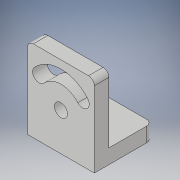
# Autodesk Inventor part: RotateLBracket
Saved by Autodesk Inventor 2019 (Build 230136000, 136)
## iProperties
Created: 2019-08-13
Part Number: RotateLBracket
Material: Generic
Document SubType Name: Modeling
Designer: aorfi
Density: 1 g/cm^3
Appearance: Default
Author: aorfi
Autodesk Inventor part; units mm, degrees
ref_plane "YZ Plane" through (0, 0, 0) normal (1, 0, 0) x (0, 1, 0)
ref_plane "XZ Plane" through (0, 0, 0) normal (0, 1, 0) x (-1, 0, 0)
ref_plane "XY Plane" through (0, 0, 0) normal (0, 0, 1) x (1, 0, 0)
sketch "Sketch1" plane through (0, 0, 0) normal (0, 0, 1) x (1, 0, 0)
  line L0 (-11.5, -14) -> (11.5, -14)
  line L1 (11.5, -14) -> (11.5, 14)
  line L2 (11.5, 14) -> (-11.5, 14)
  line L3 (-11.5, 14) -> (-11.5, -14)
  line L4 (-11.5, -14) -> (11.5, 14) construction
  line L5 (11.5, -14) -> (-11.5, 14) construction
  point P0 (0, 0)
  dimension "d0" = 23
  dimension "d1" = 28
  constraints: 12 end point, 2 midpoint, 2 parallel, 1 horizontal, 1 perpendicular
  measures "d0" distance of L1.end L2.end
  measures "d1" distance of L0.end L1.end
extrude "Extrusion1" add sketch "Sketch1" along normal mid plane 5
sketch "Sketch2" plane through (0, 0, -2.5) normal (0, 0, -1) x (-1, 0, 0)
  line L0 (11.5, -14) -> (-11.5, -14) projected
  line L1 (-11.5, -14) -> (11.5, -14)
  line L2 (11.5, -14) -> (11.5, -9)
  line L3 (11.5, -9) -> (-11.5, -9)
  line L4 (-11.5, -9) -> (-11.5, -14)
  line L5 (11.5, -14) -> (11.5, 14) projected
  point P0 (0, 0)
  dimension "d4" = 5
  constraints: 8 end point, 2 parallel, 1 collinear, 1 horizontal, 1 perpendicular
  measures "d4" distance between parallel lines of L0 L3
extrude "Extrusion2" add sketch "Sketch2" along normal blind 15
sketch "Sketch3" plane through (-11.5, -9, -2.5) normal (0, 1, 0) x (1, 0, 0)
  line L0 (0, 0) -> (0, 15) projected
  line L1 (0, 15) -> (23, 15) projected
  point P0 (11.5, -2.5)
  point P1 (11.5, 7.5)
  point P2 (0, 7.5)
  point P3 (11.5, 15)
  constraints: 2 midpoint, 1 horizontal alignment, 1 vertical alignment
hole "Hole1" at (0, -9, -10) direction (0, -1, 0) diameter 4.496 end through all clearance for "Flat Head Machine Screw (82)" size "#8" standard "Ansi Unified Screw Threads"
sketch "Sketch4" plane through (0, 0, -2.5) normal (0, 0, -1) x (-1, 0, 0)
  line L0 (11.5, 14) -> (-11.5, 14) projected
  line L1 (11.5, -9) -> (-11.5, -9) projected
  point P0 (0, 0)
  point P1 (0, -1)
  point P2 (0, 14)
  dimension "d14" = 8
  constraints: 1 midpoint, 1 vertical alignment
  measures "d14" distance from line of L1 point (0, -1)
hole "Hole2" at (0, -1, -2.5) direction (0, 0, 1) diameter 4.496 end through all clearance for "Flat Head Machine Screw (82)" size "#8" standard "Ansi Unified Screw Threads"
sketch "Sketch5" plane through (0, 0, -2.5) normal (0, 0, -1) x (-1, 0, 0)
  circle A0 centre (0, -1) radius 10 construction
  arc A1 (-9.186, 7.1013) -> (-5.814, 4.1275) centre (-7.5, 5.6144) ccw
  arc A2 (5.814, 4.1275) -> (9.186, 7.1013) centre (7.5, 5.6144) ccw
  arc A3 (9.186, 7.1013) -> (-9.186, 7.1013) centre (0, -1) ccw
  arc A4 (5.814, 4.1275) -> (-5.814, 4.1275) centre (0, -1) ccw
  line L0 (-7.5, 5.6144) -> (7.5, 5.6144) construction
  line L1 (-11.5, 14) -> (-11.5, -9) construction
  circle A5 centre (0, -1) radius 2.248 projected
  point P0 (0, 5.6144)
  dimension "d22" = 20
  dimension "d23" = 4.496
  dimension "d24" = 4
  constraints: 11 point on circle, 5 centre point, 4 tangent, 3 concentric, 2 coincident, 2 end point, 1 equal radius, 1 horizontal, 1 midpoint, 1 vertical alignment
  measures "d22" diameter of A0
  measures "d23" diameter of A1
  measures "d24" distance from line of L1 A1.centre
extrude "Extrusion3" cut sketch "Sketch5" against normal through all contours A3 A2 A4 A1
fillet "Fillet1" radius 2 4 edges at (11.5, 14, 0) (-11.5, 14, 0) (11.5, -11.5, -17.5) (-11.5, -11.5, -17.5)
body "Solid1"
